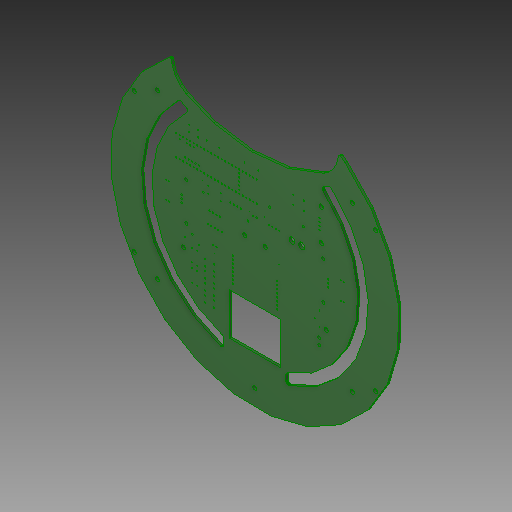
# Autodesk Inventor part: Board 3 Teensy.brd_Outline
Saved by Autodesk Inventor 2017 (Build 210142000, 142)
## iProperties
Created: 2019-06-13
Part Number: Board 3 Teensy.brd_Outline
Material: Generic
Document SubType Name: Modeling
Designer: Marc
Density: 1 g/cm^3
Appearance: Board Outline
Author: Marc
Autodesk Inventor part; units mm, degrees
ref_plane "YZ Plane" through (0, 0, 0) normal (1, 0, 0) x (0, 1, 0)
ref_plane "XZ Plane" through (0, 0, 0) normal (0, 1, 0) x (-1, 0, 0)
ref_plane "XY Plane" through (0, 0, 0) normal (0, 0, 1) x (1, 0, 0)
sketch "Sketch1" plane through (0, 0, 0) normal (0, 0, 1) x (1, 0, 0)
  line L0 (-22.4968, -72.8805) -> (-22.4968, -76.6703)
  line L1 (-22.4968, -76.6703) -> (-22.565, -77.188)
  line L2 (-22.565, -77.188) -> (-22.7648, -77.6703)
  line L3 (-22.7648, -77.6703) -> (-23.0827, -78.0845)
  line L4 (-23.0827, -78.0845) -> (-23.4969, -78.4024)
  line L5 (-23.4969, -78.4024) -> (-23.9793, -78.6022)
  line L6 (-23.9793, -78.6022) -> (-24.497, -78.6703)
  line L7 (-24.497, -78.6703) -> (-25.0146, -78.6021)
  line L8 (-25.0146, -78.6021) -> (-25.052, -78.5917)
  line L9 (-25.052, -78.5917) -> (-44.5395, -69.4293)
  line L10 (-44.5395, -69.4293) -> (-60.9917, -55.5354)
  line L11 (-60.9917, -55.5354) -> (-73.2872, -37.8567)
  line L12 (-73.2872, -37.8567) -> (-80.5882, -17.5981)
  line L13 (-80.5882, -17.5981) -> (-82.3971, 3.8598)
  line L14 (-82.3971, 3.8598) -> (-78.5907, 25.0548)
  line L15 (-78.5907, 25.0548) -> (-69.4283, 44.5423)
  line L16 (-69.4283, 44.5423) -> (-55.6939, 60.8489)
  line L17 (-55.6939, 60.8489) -> (-55.2443, 61.1144)
  line L18 (-55.2443, 61.1144) -> (-54.7414, 61.2546)
  line L19 (-54.7414, 61.2546) -> (-54.2193, 61.2598)
  line L20 (-54.2193, 61.2598) -> (-53.7136, 61.1297)
  line L21 (-53.7136, 61.1297) -> (-53.5093, 61.0337)
  line L22 (-53.5093, 61.0337) -> (-50.1523, 59.2908)
  line L23 (-50.1523, 59.2908) -> (-49.7193, 58.999)
  line L24 (-49.7193, 58.999) -> (-49.3766, 58.6052)
  line L25 (-49.3766, 58.6052) -> (-49.1475, 58.136)
  line L26 (-49.1475, 58.136) -> (-49.0477, 57.6235)
  line L27 (-49.0477, 57.6235) -> (-49.0839, 57.1027)
  line L28 (-49.0839, 57.1027) -> (-49.2536, 56.6089)
  line L29 (-49.2536, 56.6089) -> (-49.5454, 56.176)
  line L30 (-49.5454, 56.176) -> (-49.7161, 56.0048)
  line L31 (-49.7161, 56.0048) -> (-62.5174, 41.2299)
  line L32 (-62.5174, 41.2299) -> (-71.0584, 23.6452)
  line L33 (-71.0584, 23.6452) -> (-74.7572, 4.4492)
  line L34 (-74.7572, 4.4492) -> (-73.3616, -15.0501)
  line L35 (-73.3616, -15.0501) -> (-66.9668, -33.5238)
  line L36 (-66.9668, -33.5238) -> (-56.0085, -49.7129)
  line L37 (-56.0085, -49.7129) -> (-41.2336, -62.5142)
  line L38 (-41.2336, -62.5142) -> (-23.8596, -70.9847)
  line L39 (-23.8596, -70.9847) -> (-23.3907, -71.2143)
  line L40 (-23.3907, -71.2143) -> (-22.9971, -71.5573)
  line L41 (-22.9971, -71.5573) -> (-22.7057, -71.9906)
  line L42 (-22.7057, -71.9906) -> (-22.5364, -72.4845)
  line L43 (-22.5364, -72.4845) -> (-22.4968, -72.8805)
  line L44 (24.8977, -78.6406) -> (24.3768, -78.6759)
  line L45 (24.3768, -78.6759) -> (23.8645, -78.5752)
  line L46 (23.8645, -78.5752) -> (23.3958, -78.3453)
  line L47 (23.3958, -78.3453) -> (23.0025, -78.002)
  line L48 (23.0025, -78.002) -> (22.7114, -77.5685)
  line L49 (22.7114, -77.5685) -> (22.5425, -77.0745)
  line L50 (22.5425, -77.0745) -> (22.5032, -76.6799)
  line L51 (22.5032, -76.6799) -> (22.5032, -72.8782)
  line L52 (22.5032, -72.8782) -> (22.5713, -72.3606)
  line L53 (22.5713, -72.3606) -> (22.7711, -71.8783)
  line L54 (22.7711, -71.8783) -> (23.0889, -71.4641)
  line L55 (23.0889, -71.4641) -> (23.503, -71.1462)
  line L56 (23.503, -71.1462) -> (23.8658, -70.9825)
  line L57 (23.8658, -70.9825) -> (41.4243, -62.3867)
  line L58 (41.4243, -62.3867) -> (56.1598, -49.5394)
  line L59 (56.1598, -49.5394) -> (67.068, -33.3159)
  line L60 (67.068, -33.3159) -> (73.4057, -14.822)
  line L61 (73.4057, -14.822) -> (74.7408, 4.682)
  line L62 (74.7408, 4.682) -> (70.9824, 23.867)
  line L63 (70.9824, 23.867) -> (62.3866, 41.4255)
  line L64 (62.3866, 41.4255) -> (49.7154, 56.0051)
  line L65 (49.7154, 56.0051) -> (49.3735, 56.3997)
  line L66 (49.3735, 56.3997) -> (49.1454, 56.8693)
  line L67 (49.1454, 56.8693) -> (49.0467, 57.382)
  line L68 (49.0467, 57.382) -> (49.084, 57.9028)
  line L69 (49.084, 57.9028) -> (49.2548, 58.3962)
  line L70 (49.2548, 58.3962) -> (49.5475, 58.8285)
  line L71 (49.5475, 58.8285) -> (49.9421, 59.1704)
  line L72 (49.9421, 59.1704) -> (50.1516, 59.2911)
  line L73 (50.1516, 59.2911) -> (53.5122, 61.0359)
  line L74 (53.5122, 61.0359) -> (54, 61.2222)
  line L75 (54, 61.2222) -> (54.5193, 61.2758)
  line L76 (54.5193, 61.2758) -> (55.0349, 61.1933)
  line L77 (55.0349, 61.1933) -> (55.5115, 60.9801)
  line L78 (55.5115, 60.9801) -> (55.661, 60.8785)
  line L79 (55.661, 60.8785) -> (69.5212, 44.3989)
  line L80 (69.5212, 44.3989) -> (78.6438, 24.8936)
  line L81 (78.6438, 24.8936) -> (82.4073, 3.6918)
  line L82 (82.4073, 3.6918) -> (80.5551, -17.7616)
  line L83 (80.5551, -17.7616) -> (73.2134, -38.0047)
  line L84 (73.2134, -38.0047) -> (60.8826, -55.6578)
  line L85 (60.8826, -55.6578) -> (44.4031, -69.5179)
  line L86 (44.4031, -69.5179) -> (24.8977, -78.6406)
  line L87 (-18.4968, -39.9324) -> (18.5032, -39.9324)
  line L88 (18.5032, -39.9324) -> (18.5032, -70.4324)
  line L89 (18.5032, -70.4324) -> (-18.4968, -70.4324)
  line L90 (-18.4968, -70.4324) -> (-18.4968, -39.9324)
  line L91 (-60.7504, 83.7894) -> (-60.8105, 84.0434)
  line L92 (-60.8105, 84.0434) -> (-60.9343, 84.2733)
  line L93 (-60.9343, 84.2733) -> (-61.1134, 84.4632)
  line L94 (-61.1134, 84.4632) -> (-61.3355, 84.6003)
  line L95 (-61.3355, 84.6003) -> (-61.5856, 84.6753)
  line L96 (-61.5856, 84.6753) -> (-61.8465, 84.683)
  line L97 (-61.8465, 84.683) -> (-62.1006, 84.6229)
  line L98 (-62.1006, 84.6229) -> (-62.3304, 84.4991)
  line L99 (-62.3304, 84.4991) -> (-62.339, 84.4928)
  line L100 (-62.339, 84.4928) -> (-82.0829, 65.4793)
  line L101 (-82.0829, 65.4793) -> (-96.2331, 42.0037)
  line L102 (-96.2331, 42.0037) -> (-103.8251, 15.6656)
  line L103 (-103.8251, 15.6656) -> (-104.3417, -11.7401)
  line L104 (-104.3417, -11.7401) -> (-97.7475, -38.3455)
  line L105 (-97.7475, -38.3455) -> (-84.4921, -62.3378)
  line L106 (-84.4921, -62.3378) -> (-65.4786, -82.0817)
  line L107 (-65.4786, -82.0817) -> (-42.0029, -96.2319)
  line L108 (-42.0029, -96.2319) -> (-15.6648, -103.8239)
  line L109 (-15.6648, -103.8239) -> (11.7408, -104.3405)
  line L110 (11.7408, -104.3405) -> (38.3463, -97.7464)
  line L111 (38.3463, -97.7464) -> (62.3385, -84.4909)
  line L112 (62.3385, -84.4909) -> (82.0825, -65.4774)
  line L113 (82.0825, -65.4774) -> (96.2326, -42.0018)
  line L114 (96.2326, -42.0018) -> (103.8247, -15.6637)
  line L115 (103.8247, -15.6637) -> (104.3412, 11.742)
  line L116 (104.3412, 11.742) -> (97.7471, 38.3475)
  line L117 (97.7471, 38.3475) -> (84.4916, 62.3397)
  line L118 (84.4916, 62.3397) -> (65.4782, 82.0836)
  line L119 (65.4782, 82.0836) -> (62.3379, 84.4932)
  line L120 (62.3379, 84.4932) -> (62.1094, 84.6195)
  line L121 (62.1094, 84.6195) -> (61.856, 84.6823)
  line L122 (61.856, 84.6823) -> (61.595, 84.6773)
  line L123 (61.595, 84.6773) -> (61.3442, 84.605)
  line L124 (61.3442, 84.605) -> (61.1206, 84.4703)
  line L125 (61.1206, 84.4703) -> (60.9395, 84.2822)
  line L126 (60.9395, 84.2822) -> (60.8133, 84.0537)
  line L127 (60.8133, 84.0537) -> (60.7505, 83.8003)
  line L128 (60.7505, 83.8003) -> (60.7494, 83.7899)
  line L129 (60.7494, 83.7899) -> (59.5029, 78.525)
  line L130 (59.5029, 78.525) -> (56.9362, 73.7622)
  line L131 (56.9362, 73.7622) -> (53.2243, 69.8259)
  line L132 (53.2243, 69.8259) -> (50.001, 67.6673)
  line L133 (50.001, 67.6673) -> (24.4028, 57.8712)
  line L134 (24.4028, 57.8712) -> (-2.8586, 55.0341)
  line L135 (-2.8586, 55.0341) -> (-29.9254, 59.3495)
  line L136 (-29.9254, 59.3495) -> (-50.0023, 67.665)
  line L137 (-50.0023, 67.665) -> (-54.3828, 70.8411)
  line L138 (-54.3828, 70.8411) -> (-57.7921, 75.0427)
  line L139 (-57.7921, 75.0427) -> (-59.9978, 79.9836)
  line L140 (-59.9978, 79.9836) -> (-60.7504, 83.7894)
  circle A0 centre (-36.27, -29.49) radius 0.51
  circle A1 centre (-29.77, -29.49) radius 0.51
  circle A2 centre (-36.27, -34.01) radius 0.51
  circle A3 centre (-29.77, -34.01) radius 0.51
  circle A4 centre (-36.27, -37.11) radius 0.51
  circle A5 centre (-29.77, -37.11) radius 0.51
  circle A6 centre (-36.27, -41.63) radius 0.51
  circle A7 centre (-29.77, -41.63) radius 0.51
  circle A8 centre (-36.27, -44.73) radius 0.51
  circle A9 centre (-29.77, -44.73) radius 0.51
  circle A10 centre (-36.27, -49.25) radius 0.51
  circle A11 centre (-29.77, -49.25) radius 0.51
  circle A12 centre (-36.27, -52.35) radius 0.51
  circle A13 centre (-29.77, -52.35) radius 0.51
  circle A14 centre (-36.27, -56.87) radius 0.51
  circle A15 centre (-29.77, -56.87) radius 0.51
  circle A16 centre (62.48, -6.35) radius 0.405
  circle A17 centre (64.52, -6.35) radius 0.405
  circle A18 centre (62.48, 6.35) radius 0.405
  circle A19 centre (64.52, 6.35) radius 0.405
  circle A20 centre (-62.48, 6.35) radius 0.405
  circle A21 centre (-64.52, 6.35) radius 0.405
  circle A22 centre (-62.48, -6.35) radius 0.405
  circle A23 centre (-64.52, -6.35) radius 0.405
  circle A24 centre (-16.13, -34.93) radius 0.51
  circle A25 centre (-16.13, -32.39) radius 0.51
  circle A26 centre (-16.13, -29.85) radius 0.51
  circle A27 centre (-16.13, -27.31) radius 0.51
  circle A28 centre (-16.13, -24.77) radius 0.51
  circle A29 centre (-16.13, -22.23) radius 0.51
  circle A30 centre (-16.13, -19.69) radius 0.51
  circle A31 centre (-16.13, -17.15) radius 0.51
  circle A32 centre (16.13, -34.93) radius 0.51
  circle A33 centre (16.13, -32.39) radius 0.51
  circle A34 centre (16.13, -29.85) radius 0.51
  circle A35 centre (16.13, -27.31) radius 0.51
  circle A36 centre (16.13, -24.77) radius 0.51
  circle A37 centre (16.13, -22.23) radius 0.51
  circle A38 centre (16.13, -19.69) radius 0.51
  circle A39 centre (16.13, -17.15) radius 0.51
  circle A40 centre (46.93, 30.48) radius 0.51
  circle A41 centre (46.93, 33.02) radius 0.51
  circle A42 centre (46.93, 35.56) radius 0.51
  circle A43 centre (46.93, 38.1) radius 0.51
  circle A44 centre (27.94, 36.83) radius 0.405
  circle A45 centre (35.56, 36.83) radius 0.405
  circle A46 centre (27.94, 43.18) radius 0.405
  circle A47 centre (35.56, 43.18) radius 0.405
  circle A48 centre (53.34, 0) radius 0.51
  circle A49 centre (53.34, -2.54) radius 0.51
  circle A50 centre (53.34, 2.54) radius 0.51
  circle A51 centre (-53.34, 0) radius 0.51
  circle A52 centre (-53.34, 2.54) radius 0.51
  circle A53 centre (-53.34, -2.54) radius 0.51
  circle A54 centre (-33.02, 2.54) radius 0.51
  circle A55 centre (-30.48, 2.54) radius 0.51
  circle A56 centre (-27.94, 2.54) radius 0.51
  circle A57 centre (-25.4, 2.54) radius 0.51
  circle A58 centre (10.16, 15.24) radius 0.51
  circle A59 centre (12.7, 15.24) radius 0.51
  circle A60 centre (15.24, 15.24) radius 0.51
  circle A61 centre (17.78, 15.24) radius 0.51
  circle A62 centre (-34.29, -6.35) radius 0.51
  circle A63 centre (-31.75, -6.35) radius 0.51
  circle A64 centre (-29.21, -6.35) radius 0.51
  circle A65 centre (-26.67, -6.35) radius 0.51
  circle A66 centre (-24.13, -6.35) radius 0.51
  circle A67 centre (-27.94, -17.78) radius 0.51
  circle A68 centre (-30.48, -17.78) radius 0.51
  circle A69 centre (-17.78, 15.24) radius 0.51
  circle A70 centre (-15.24, 15.24) radius 0.51
  circle A71 centre (-12.7, 15.24) radius 0.51
  circle A72 centre (-10.16, 15.24) radius 0.51
  circle A73 centre (1.27, 15.24) radius 0.51
  circle A74 centre (-1.27, 15.24) radius 0.51
  circle A75 centre (46.99, -30.48) radius 0.405
  circle A76 centre (46.99, -20.32) radius 0.405
  circle A77 centre (-50.8, -22.86) radius 0.405
  circle A78 centre (-40.64, -22.86) radius 0.405
  circle A79 centre (-24.64, 17.78) radius 0.405
  circle A80 centre (-33.78, 17.78) radius 0.405
  circle A81 centre (-24.64, 12.7) radius 0.405
  circle A82 centre (-33.78, 12.7) radius 0.405
  circle A83 centre (-25.91, 45.72) radius 0.405
  circle A84 centre (-35.05, 45.72) radius 0.405
  circle A85 centre (-41.91, -27.18) radius 0.405
  circle A86 centre (-41.91, -36.32) radius 0.405
  circle A87 centre (-45.72, -27.18) radius 0.405
  circle A88 centre (-45.72, -36.32) radius 0.405
  circle A89 centre (-41.91, -39.88) radius 0.405
  circle A90 centre (-41.91, -49.02) radius 0.405
  circle A91 centre (-45.72, -39.88) radius 0.405
  circle A92 centre (-45.72, -49.02) radius 0.405
  circle A93 centre (2.54, 45.72) radius 0.405
  circle A94 centre (-7.62, 45.72) radius 0.405
  circle A95 centre (-47.7, 49.25) radius 0.51
  circle A96 centre (-41.2, 49.25) radius 0.51
  circle A97 centre (-47.7, 44.73) radius 0.51
  circle A98 centre (-41.2, 44.73) radius 0.51
  circle A99 centre (10.61, 26.67) radius 0.75
  circle A100 centre (35.11, 26.67) radius 0.75
  circle A101 centre (26.98, 13.97) radius 2.25
  circle A102 centre (33.98, 13.97) radius 2.25
  circle A103 centre (-54.61, 24.13) radius 0.485
  circle A104 centre (-52.07, 24.13) radius 0.485
  circle A105 centre (-49.53, 24.13) radius 0.485
  circle A106 centre (-46.99, 24.13) radius 0.485
  circle A107 centre (-52.07, 39.37) radius 0.485
  circle A108 centre (-21.59, 24.13) radius 0.485
  circle A109 centre (-11.43, 29.21) radius 0.485
  circle A110 centre (-44.45, 24.13) radius 0.485
  circle A111 centre (-41.91, 24.13) radius 0.485
  circle A112 centre (-39.37, 24.13) radius 0.485
  circle A113 centre (-36.83, 24.13) radius 0.485
  circle A114 centre (-34.29, 24.13) radius 0.485
  circle A115 centre (-31.75, 24.13) radius 0.485
  circle A116 centre (-29.21, 24.13) radius 0.485
  circle A117 centre (-26.67, 24.13) radius 0.485
  circle A118 centre (-24.13, 24.13) radius 0.485
  circle A119 centre (-24.13, 39.37) radius 0.485
  circle A120 centre (-26.67, 39.37) radius 0.485
  circle A121 centre (-29.21, 39.37) radius 0.485
  circle A122 centre (-31.75, 39.37) radius 0.485
  circle A123 centre (-34.29, 39.37) radius 0.485
  circle A124 centre (-36.83, 39.37) radius 0.485
  circle A125 centre (-39.37, 39.37) radius 0.485
  circle A126 centre (-41.91, 39.37) radius 0.485
  circle A127 centre (-44.45, 39.37) radius 0.485
  circle A128 centre (-46.99, 39.37) radius 0.485
  circle A129 centre (-49.53, 39.37) radius 0.485
  circle A130 centre (-19.05, 24.13) radius 0.485
  circle A131 centre (-16.51, 24.13) radius 0.485
  circle A132 centre (-13.97, 24.13) radius 0.485
  circle A133 centre (-11.43, 24.13) radius 0.485
  circle A134 centre (-8.89, 24.13) radius 0.485
  circle A135 centre (-6.35, 24.13) radius 0.485
  circle A136 centre (-3.81, 24.13) radius 0.485
  circle A137 centre (-1.27, 24.13) radius 0.485
  circle A138 centre (1.27, 24.13) radius 0.485
  circle A139 centre (1.27, 39.37) radius 0.485
  circle A140 centre (-1.27, 39.37) radius 0.485
  circle A141 centre (-3.81, 39.37) radius 0.485
  circle A142 centre (-6.35, 39.37) radius 0.485
  circle A143 centre (-8.89, 39.37) radius 0.485
  circle A144 centre (-11.43, 39.37) radius 0.485
  circle A145 centre (-13.97, 39.37) radius 0.485
  circle A146 centre (-46.99, 36.83) radius 0.485
  circle A147 centre (-44.45, 36.83) radius 0.485
  circle A148 centre (-16.51, 39.37) radius 0.485
  circle A149 centre (-19.05, 39.37) radius 0.485
  circle A150 centre (-45.72, 27.3) radius 0.485
  circle A151 centre (-48.26, 27.3) radius 0.485
  circle A152 centre (-54.61, 39.37) radius 0.485
  circle A153 centre (-49.53, 36.83) radius 0.485
  circle A154 centre (-57.15, 24.13) radius 0.485
  circle A155 centre (-21.59, 39.37) radius 0.485
  circle A156 centre (-43.18, 27.3) radius 0.485
  circle A157 centre (-40.64, 27.3) radius 0.485
  circle A158 centre (-11.43, 31.75) radius 0.485
  circle A159 centre (-50.8, 27.3) radius 0.485
  circle A160 centre (-11.43, 34.29) radius 0.485
  circle A161 centre (-11.43, 36.83) radius 0.485
  circle A162 centre (-11.43, 26.67) radius 0.485
  circle A163 centre (-57.15, 39.37) radius 0.485
  circle A164 centre (-54.61, 36.83) radius 0.485
  circle A165 centre (46.78, -37.46) radius 1.05
  circle A166 centre (46.78, -42.16) radius 1.05
  circle A167 centre (-87.6848, 50.6254) radius 1.5
  circle A168 centre (-70.8591, 59.4581) radius 1.5
  circle A169 centre (70.8591, 59.4581) radius 1.5
  circle A170 centre (87.6848, 50.6254) radius 1.5
  circle A171 centre (7.4999, 0) radius 1.5
  circle A172 centre (-7.4999, 0) radius 1.5
  circle A173 centre (-51.8178, -29.9156) radius 1.5
  circle A174 centre (-87.6853, -50.6246) radius 1.5
  circle A175 centre (-70.8591, -59.4576) radius 1.5
  circle A176 centre (0, -92.4998) radius 1.5
  circle A177 centre (70.8591, -59.4576) radius 1.5
  circle A178 centre (87.6853, -50.6246) radius 1.5
  circle A179 centre (51.8178, -29.9156) radius 1.5
  circle A180 centre (48.2, 45.72) radius 1.651
  circle A181 centre (48.2, 22.86) radius 1.651
  circle A182 centre (-37.5, 12) radius 0.6985
  circle A183 centre (-5, 10) radius 0.6985
  circle A184 centre (-45.5, -18.5) radius 0.6985
  circle A185 centre (-38, 19) radius 0.175
  circle A186 centre (-4, 16.5) radius 0.175
  circle A187 centre (49.8, -13.65) radius 1.175
  circle A188 centre (49.8, 13.65) radius 1.175
  circle A189 centre (-49.8, 13.65) radius 1.175
  circle A190 centre (-49.8, -13.65) radius 1.175
  circle A191 centre (7, 18.5) radius 0.3048
  circle A192 centre (-29.5, -22.5) radius 0.3048
  circle A193 centre (17.5, -6) radius 0.3048
  circle A194 centre (43.5, -27) radius 0.3048
  constraints: 282 end point, 195 centre point
extrude "Board 3 Teensy.brd_Outline" add sketch "Sketch1" along normal blind 1.6
body "Solid1"
